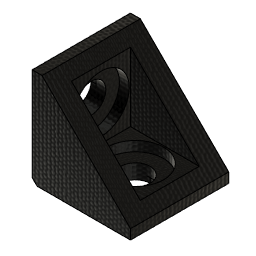
ExtrusionConnector (Autodesk Fusion 360 design; units mm, degrees)
part number: T-slot extrusion connectors
part number: CornerBracket
part number: Extrusion
Autodesk Fusion 360 part; units mm, degrees
note: some values were not read from the file. Set by a fixed rule: which sketch regions a step uses.
sketch "bracket sketch" plane through (0, 0, 0) normal (0, 1, 0) x (1, 0, 0) in component "CornerBracket"
  line L0 (0, 0) -> (0, -20)
  line L1 (0, 0) -> (30, 0)
  line L2 (0, -20) -> (2, -20)
  line L3 (4, -4) -> (4, -27.8333)
  line L4 (4, -4) -> (27.8333, -4)
  line L5 (0, 0) -> (-1, 0)
  line L6 (-1, 0) -> (-1, -20)
  line L7 (-1, -20) -> (0, -20)
  line L8 (0, -20) -> (0, 0)
  line L9 (0, 0) -> (30, 0)
  line L10 (0, 0) -> (20, 0)
  line L11 (0, 0) -> (20, 0)
  line L12 (20, 0) -> (20, 1)
  line L13 (20, 1) -> (0, 1)
  line L14 (0, 1) -> (0, 0)
  line L15 (20, 0) -> (20, -2)
  line L16 (20, -2) -> (2, -20)
  point P0 (15.9167, -4)
  point P1 (4, -15.9167)
  dimension "d14" = 20
  dimension "d16" = 2
  dimension "d22" = 4
  dimension "d24" = 4
  dimension "d62" = 20
  dimension "d63" = 1
  dimension "d64" = 20
  dimension "d77" = 20
  dimension "d78" = 1
  dimension "d79" = 2
  constraint coincident L0.start L1.start
  constraint vertical L0
  constraint horizontal L1
  constraint perpendicular L0 L2
  constraint vertical L3
  constraint perpendicular L3 L4
  constraint horizontal L5
  constraint vertical L6
  constraint horizontal L7
  constraint vertical L8
  constraint horizontal L9
  constraint horizontal L10
  constraint coincident L4 P0
  constraint midpoint L4 P0
  constraint midpoint L3 P1
  constraint horizontal L11
  constraint vertical L12
  constraint horizontal L13
  constraint vertical L14
  constraint vertical L15
  measures "d14" distance of L0.start L0.end
  measures "d16" distance of L0.end L2.end
  measures "d22" distance of L0 L3
  measures "d24" distance of L1 L4.end
  measures "d62" distance of L0.start L0.end
  measures "d63" distance of L0.start L5.end
  measures "d64" distance of L0.start L10.end
  measures "d77" distance of L0.start L10.end
  measures "d78" distance of L0.start L13.end
  measures "d79" distance of L10.end L15.end
extrude "Extrude6" add sketch "bracket sketch" along normal mid plane 20 contours L0 L1 L2 L3 L4 L8 L9 L10 L11 L15 L16 makes body 1 in component "CornerBracket"
extrude "Extrude7" add sketch "bracket sketch" along normal blind 4 from surface at -10 contours L3 L4 L16 bodies 1 in component "CornerBracket"
extrude "Extrude8" add sketch "bracket sketch" against normal blind 4 from surface at 10 contours L3 L4 L16 bodies 1 in component "CornerBracket"
extrude "Extrude10" add sketch "bracket sketch" along normal mid plane 6 contours L1 L9 L10 L11 L12 L13 L14 | L0 L5 L6 L7 L8 bodies 1 in component "CornerBracket"
hole "Hole1" at (4, 0, 11) direction (-1, 0, 0) diameter 6 end through all counterbore diameter 11.5 counterbore depth 2 bodies 1 in component "CornerBracket"
hole "Hole2" at (11, 0, 4) direction (0, 0, -1) diameter 6 end through all counterbore diameter 11.5 counterbore depth 2 bodies 1 in component "CornerBracket"
chamfer "Chamfer2" distance 1 angle 45 6 edges at (-1, 0, 0) (0, 0, -1) (0, -6.5, 0) (0, 6.5, 0) (-1, 0, 20) (20, 0, -1) on bodies 1 in component "CornerBracket"
imported_body "Base Feature1" makes body 2 in component "5537T736"
sketch "endcap sketch" plane through (0, 0, 0) normal (1, 0, 0) x (0, 1, 0) in component "EndCap"
  line L0 (-10, 10) -> (10, 10)
  line L1 (10, 10) -> (10, -10)
  line L2 (10, -10) -> (-10, -10)
  line L3 (-10, -10) -> (-10, 10)
  line L4 (-10, 10) -> (10, -10) construction
  line L5 (10, 10) -> (-10, -10) construction
  line L6 (9, -9) -> (-9, -9)
  line L7 (-9, -9) -> (-9, 9)
  line L8 (-9, 9) -> (9, 9)
  line L9 (9, 9) -> (9, -9)
  line L10 (9, -9) -> (-9, 9) construction
  line L11 (-9, -9) -> (9, 9) construction
  dimension "d88" = 20
  dimension "d89" = 20
  dimension "d90" = 18
  dimension "d91" = 18
  constraint perpendicular L0 L1
  constraint parallel L0 L2
  constraint parallel L1 L3
  constraint horizontal L0
  constraint coincident L4 origin
  constraint coincident L5 origin
  constraint perpendicular L6 L7
  constraint parallel L6 L8
  constraint parallel L7 L9
  constraint horizontal L6
  constraint coincident L10 origin
  constraint coincident L11 origin
  measures "d88" distance of L0.end L1.end
  measures "d89" distance of L1.end L2.end
  measures "d90" distance of L7.end L8.end
  measures "d91" distance of L6.end L7.end
component "CornerBracket" placed x (1, 0, 0) y (0, 1, 0) z (0, 0, 1) at (0, 0, 0)
component "Extrusion" placed x (1, 0, 0) y (0, 1, 0) z (0, 0, 1) at (0, 0, 0)
component "EndCap" placed x (1, 0, 0) y (0, 1, 0) z (0, 0, 1) at (0, 0, 0)
component "Component" placed x (1, 0, 0) y (0, 1, 0) z (0, 0, 1) at (0, 0, 0) in component "5537T736"
hidden bodies 2
equation "extrusionSize = 20 mm" comment "use 30 for 30x30 extrusions"
equation "bracketWall = 4 mm"
equation "screwHeadWidth = 11.5 mm"
equation "screwThreadSize = 6 mm"
equation "gapFit = 0.15 mm"
equation "bracketWidth = extrusionSize"
equation "bracketHeight = extrusionSize"
equation "d14 = bracketHeight"
equation "d16 = bracketWall / 2"
equation "d22 = bracketWall"
equation "d24 = bracketWall"
equation "d34 = extrusionSize / 2"
equation "d36 = bracketWall"
equation "d38 = extrusionSize / 2"
equation "d39 = -bracketWall"
equation "d44 = -extrusionSize / 2"
equation "screwHeadSink = 2 mm"
equation "extrusionSlot = 6 mm"
equation "extrusionWall = 2 mm"
equation "d62 = extrusionSize"
equation "d63 = extrusionWall / 2"
equation "d64 = extrusionSize"
equation "d73 = screwThreadSize"
equation "d75 = screwHeadSink"
equation "d76 = screwHeadWidth"
equation "d77 = bracketWidth"
equation "d78 = extrusionWall / 2"
equation "d79 = bracketWall / 2"
equation "d81 = screwThreadSize"
equation "d83 = screwHeadSink"
equation "d84 = screwHeadWidth"
equation "d85 = extrusionSlot"
equation "d87 = extrusionWall / 2"
equation "d88 = extrusionSize"
equation "d89 = extrusionSize"
equation "d90 = extrusionSize - extrusionWall"
equation "d91 = extrusionSize - extrusionWall"
named bodies: "bracket body"
